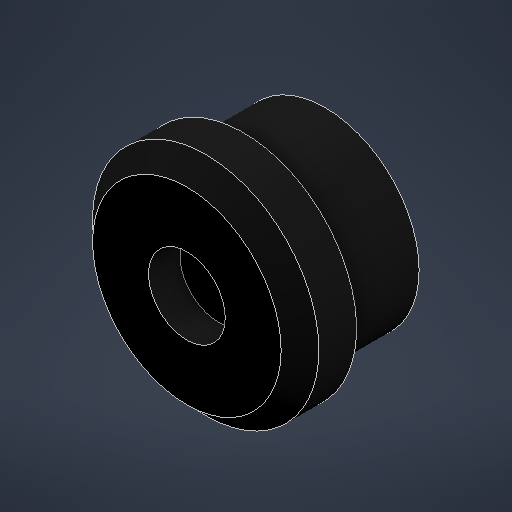
# Autodesk Inventor part: encoder_magnet_holder
Saved by Autodesk Inventor 2026.1 (Build 301233000, 233)
## iProperties
Created: 2026-04-27
Part Number: encoder_magnet_holder
Material: PET Plastic
Document SubType Name: Modeling
Designer: aaron
Density: 1.541 g/cm^3
Appearance: Polycarbonate - Clear
Author: aaron
Autodesk Inventor part; units mm, degrees
ref_plane "YZ Plane" through (0, 0, 0) normal (1, 0, 0) x (0, 1, 0)
ref_plane "XZ Plane" through (0, 0, 0) normal (0, 1, 0) x (-1, 0, 0)
ref_plane "XY Plane" through (0, 0, 0) normal (0, 0, 1) x (1, 0, 0)
sketch "Sketch1" plane through (0, 0, 0) normal (0, 0, 1) x (1, 0, 0)
  circle A0 centre (0, 0) radius 9
  dimension "d0" = 18
  constraints: 1 centre point, 1 coincident
  measures "d0" diameter of A0
extrude "Extrusion1" add sketch "Sketch1" along normal blind 4
sketch "Sketch3" plane through (0, 0, 4) normal (0, 0, 1) x (1, 0, 0)
  circle A0 centre (0, 0) radius 3.05
  dimension "d5" = 6.1
  constraints: 1 centre point, 1 coincident
  measures "d5" diameter of A0
extrude "Extrusion3" cut sketch "Sketch3" against normal blind 2.5
sketch "Sketch4" plane through (0, 0, 0) normal (0, 0, -1) x (-1, 0, 0)
  circle A0 centre (0, 0) radius 9 projected
  circle A1 centre (0, 0) radius 7.475
  dimension "d8" = 14.95
  constraints: 1 centre point, 1 coincident
  measures "d8" diameter of A1
extrude "Extrusion4" cut sketch "Sketch4" against normal blind 3.5
sketch "Sketch5" plane through (0, 0, 4) normal (0, 0, 1) x (1, 0, 0)
  circle A0 centre (0, 0) radius 3.05 projected
  circle A1 centre (0, 0) radius 9 projected
extrude "Extrusion5" add sketch "Sketch5" along normal blind 1
sketch "Sketch6" plane through (0, 0, 5) normal (0, 0, 1) x (1, 0, 0)
  circle A0 centre (0, 0) radius 7.475 projected
  circle A1 centre (0, 0) radius 9 projected
  circle A2 centre (0, 0) radius 3.05 projected
extrude "Extrusion6" add sketch "Sketch6" along normal blind 3 contours A0 | A1
sketch "Sketch7" plane through (0, 0, 0) normal (0, 0, -1) x (-1, 0, 0)
  circle A0 centre (0, 0) radius 7.475 projected
extrude "Extrusion7" add sketch "Sketch7" along normal blind 3
sketch "Sketch8" plane through (0, 0, 1.5) normal (0, 0, 1) x (1, 0, 0)
  circle A0 centre (0, 0) radius 3.05 projected
extrude "Extrusion8" add sketch "Sketch8" along normal blind 4
chamfer "Chamfer4" distance 1.5 angle 45 1 edges at (-9, 0, 8)
body "Solid1"
